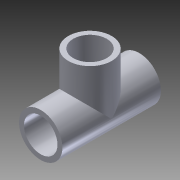
# Autodesk Inventor part: 0.5 Tee
Saved by Autodesk Inventor 2013 (Build 170138000, 138)
## iProperties
Created: 2014-07-04
Part Number: 0.5 Tee
Material: PVC-Piping
Document SubType Name: Modeling
Designer: Kyle
Density: 1 g/cm^3
Author: Kyle
Autodesk Inventor part; units mm, degrees
sketch "Sketch1" plane through (0, 0, 0) normal (0, 0, 1) x (1, 0, 0)
  circle A0 centre (0, 0) radius 13.97
  circle A1 centre (0, 0) radius 10.795
  dimension "d0" = 27.94
  dimension "d2" = 21.59
  constraints: 2 centre point, 2 coincident
  measures "d0" diameter of A0
  measures "d2" diameter of A1
extrude "Extrusion1" add sketch "Sketch1" along normal blind 63.5
ref_plane "Work Plane1" through (0, 0, 43.18) normal (0, 0, 1) x (1, 0, 0)
sketch "Sketch2" plane through (0, 0, 43.18) normal (0, 0, 1) x (1, 0, 0)
  circle A0 centre (0, 0) radius 10.414
  circle A1 centre (0, 0) radius 10.795
  dimension "d6" = 20.828
  dimension "d9" = 21.59
  constraints: 2 centre point, 2 coincident
  measures "d6" diameter of A0
  measures "d9" diameter of A1
extrude "Extrusion2" add sketch "Sketch2" against normal blind 28.829
sketch "Sketch3" plane through (0, 0, 63.5) normal (0, 0, 1) x (1, 0, 0)
  circle A0 centre (0, 0) radius 10.795 projected
  circle A1 centre (0, 0) radius 13.97 projected
  line L0 (-25.6243, 13.97) -> (27.2368, 13.97)
  constraints: 2 end point, 1 horizontal
ref_plane "Work Plane8" through (-25.6243, 32.385, 63.5) normal (0, -1, 0) x (1, 0, 0)
ref_plane "Work Plane7" through (-25.6243, 13.97, 63.5) normal (0, -1, 0) x (1, 0, 0)
sketch "Sketch10" plane through (0, 0, 0) normal (0, 0, -1) x (-1, 0, 0)
  circle A0 centre (0, 0) radius 10.795 projected
extrude "Extrusion8" cut sketch "Sketch10" against normal blind 20.32
sketch "Sketch11" plane through (-25.6243, 32.385, 63.5) normal (0, -1, 0) x (1, 0, 0)
  circle A0 centre (25.6243, -31.75) radius 13.97
  circle A1 centre (25.6243, -31.75) radius 10.795
  point P0 (25.6243, -63.5)
  dimension "d45" = 31.75
  dimension "d46" = 27.94
  dimension "d47" = 21.59
  constraints: 2 centre point, 2 coincident
  measures "d45" distance of point (25.624, -31.75) point (25.624, -63.5)
  measures "d46" diameter of A0
  measures "d47" diameter of A1
extrude "Extrusion9" add sketch "Sketch11" along normal blind 32.385
sketch "Sketch12" plane through (0, 0, 43.18) normal (0, 0, 1) x (1, 0, 0)
  arc A0 (-8.0322, 6.6284) -> (8.0322, 6.6284) centre (0, 0) ccw projected
  circle A1 centre (0, 0) radius 10.414
  constraints: 1 centre point, 1 coincident, 1 concentric
extrude "Extrusion10" cut sketch "Sketch12" against normal blind 76.2
sketch "Sketch13" plane through (0, 32.385, 31.75) normal (0, 1, 0) x (1, 0, 0)
  circle A0 centre (0, 0) radius 10.795 projected
  point P0 (0, 31.75)
extrude "Extrusion11" cut sketch "Sketch13" against normal blind 32.385
ref_plane "Work Plane9" through (0, 12.065, 31.75) normal (0, 1, 0) x (1, 0, 0)
sketch "Sketch14" plane through (0, 12.065, 31.75) normal (0, 1, 0) x (1, 0, 0)
  circle A0 centre (0, 0) radius 10.795
  circle A1 centre (0, 0) radius 10.414
  point P0 (0, 31.75)
  dimension "d55" = 21.59
  dimension "d57" = 20.828
  constraints: 2 centre point, 2 coincident
  measures "d55" diameter of A0
  measures "d57" diameter of A1
extrude "Extrusion12" add sketch "Sketch14" against normal blind 12.7
extrude "Extrusion13" cut sketch "Sketch2" along normal mid plane 76.2 contours A0
sketch "Sketch15" plane through (0, 0, 63.5) normal (0, 0, 1) x (1, 0, 0)
  circle A0 centre (0, 0) radius 10.795 projected
extrude "Extrusion14" cut sketch "Sketch15" against normal blind 20.32
sketch "Sketch16" plane through (0, 0, 0) normal (0, 0, -1) x (-1, 0, 0)
  circle A0 centre (0, 0) radius 10.795 projected
extrude "Extrusion15" cut sketch "Sketch16" against normal blind 20.32
body "Solid1"
